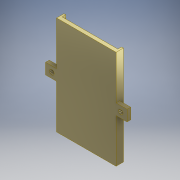
# Autodesk Inventor part: Bateria_Podkladka
Saved by Autodesk Inventor 2017 (Build 210142000, 142)
## iProperties
Created: 2016-11-21
Part Number: Bateria_Podkladka
Material: Generic
Document SubType Name: Modeling
Designer: Shichi
Density: 1 g/cm^3
Appearance: Gold - Metal
Author: Shichi
Autodesk Inventor part; units mm, degrees
ref_plane "YZ Plane" through (0, 0, 0) normal (1, 0, 0) x (0, 1, 0)
ref_plane "XZ Plane" through (0, 0, 0) normal (0, 1, 0) x (-1, 0, 0)
ref_plane "XY Plane" through (0, 0, 0) normal (0, 0, 1) x (1, 0, 0)
sketch "Sketch1" plane through (0, 0, 0) normal (0, 1, 0) x (-1, 0, 0)
  line L0 (-16.25, 27) -> (16.25, 27)
  line L1 (16.25, 27) -> (16.25, -27)
  line L2 (16.25, -27) -> (-16.25, -27)
  line L3 (-16.25, -27) -> (-16.25, 27)
  line L4 (-16.25, 27) -> (16.25, -27) construction
  line L5 (16.25, 27) -> (-16.25, -27) construction
  line L6 (16.25, 3) -> (22.25, 3)
  line L7 (22.25, 3) -> (22.25, -3)
  line L8 (22.25, -3) -> (16.25, -3)
  line L9 (16.25, -3) -> (16.25, 3)
  line L10 (-16.25, 3) -> (-22.25, 3)
  line L11 (-22.25, 3) -> (-22.25, -3)
  line L12 (-22.25, -3) -> (-16.25, -3)
  line L13 (-16.25, -3) -> (-16.25, 3)
  circle A0 centre (18.85, 0) radius 1.25
  circle A1 centre (-18.85, 0) radius 1.25
  point P0 (0, 0)
  point P1 (19.25, -3)
  point P2 (19.25, 3)
  point P3 (22.25, 0)
  point P4 (16.25, 0)
  point P5 (-22.25, 0)
  point P6 (-16.25, 0)
  dimension "d0" = 54
  dimension "d1" = 32.5
  dimension "d12" = 6
  dimension "d13" = 6
  dimension "d14" = 6
  dimension "d15" = 6
  dimension "d16" = 2.5
  dimension "d17" = 2.5
  dimension "d18" = 2.6
  dimension "d19" = 37.7
  dimension "d20" = 3
  dimension "d21" = 3
  constraints: 28 end point, 8 midpoint, 6 parallel, 3 horizontal, 3 perpendicular, 2 centre point, 2 horizontal alignment, 2 point on line, 1 vertical alignment
  measures "d0" distance of L0.end L1.end
  measures "d1" distance of L1.end L2.end
  measures "d12" distance of L6.end L7.end
  measures "d13" distance of L6.start L6.end
  measures "d14" distance of L11.end L12.end
  measures "d15" distance of L10.end L11.end
  measures "d16" diameter of A0
  measures "d17" diameter of A1
  measures "d18" distance from line of L1 A0.centre
  measures "d19" distance of A0.centre A1.centre
  measures "d20" distance from line of L6 A0.centre
  measures "d21" distance from line of L10 A1.centre
extrude "Extrusion1" add sketch "Sketch1" along normal blind 2
sketch "Sketch2" plane through (0, 2, 0) normal (0, 1, 0) x (1, 0, 0)
  line L0 (-16.25, -27) -> (16.25, -27) projected
  line L1 (-16.25, 27) -> (-16.25, -27) projected
  line L2 (16.25, 27) -> (-16.25, 27) projected
  line L3 (-16.25, -27) -> (-15.25, -27)
  line L4 (-15.25, -27) -> (-15.25, 27)
  line L5 (-15.25, 27) -> (-16.25, 27)
  line L6 (-16.25, 27) -> (-16.25, -27)
  line L7 (0, -27) -> (0, 27) construction
  line L8 (16.25, -27) -> (15.25, -27)
  line L9 (15.25, -27) -> (15.25, 27)
  line L10 (15.25, 27) -> (16.25, 27)
  line L11 (16.25, 27) -> (16.25, -27)
  point P0 (0, 0)
  dimension "d4" = 1
  dimension "d5" = 1
  constraints: 18 end point, 4 parallel, 2 horizontal, 2 midpoint, 2 perpendicular, 2 point on line
  measures "d4" distance of L0.start L3.end
  measures "d5" distance of L0.end L8.end
extrude "Extrusion2" add sketch "Sketch2" along normal blind 2 contours L1 L2 L4 L0 | L9 L2 L11 L0
body "Solid1"
